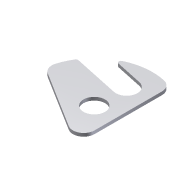
# Autodesk Inventor part: OpenROV 2_3 Dev EndCap Wire Guide
Saved by Autodesk Inventor 2012 (Build 160160000, 160)
## iProperties
Created: 2011-09-29
Part Number: OpenROV 2_3 Dev EndCap Wire Guide
Document SubType Name: Modeling
Designer: user
Density: 1 g/cm^3
Material: Default
Author: user
Autodesk Inventor part; units mm, degrees
ref_plane "YZ Plane" through (0, 0, 0) normal (1, 0, 0) x (0, 1, 0)
ref_plane "XZ Plane" through (0, 0, 0) normal (0, 1, 0) x (-1, 0, 0)
ref_plane "XY Plane" through (0, 0, 0) normal (0, 0, 1) x (1, 0, 0)
sketch "Sketch1" plane through (0, 0, 0) normal (0, 0, 1) x (1, 0, 0)
  arc A0 (-2.0957, 20.2221) -> (2.0957, 39.7779) centre (0, 30) ccw
  line L0 (2.0957, 39.7779) -> (-22.6081, 45.0726)
  line L1 (-2.0957, 20.2221) -> (-43.8855, 29.1787)
  arc A1 (12.2727, 52.5869) -> (-23.0424, 48.837) centre (0, 0) ccw
  line L2 (-47.415, 4.2576) -> (4.7008, -28.308)
  arc A2 (-46.0087, 28.2702) -> (-51.6876, 15.6331) centre (0, 0) ccw
  line L3 (20, -19.8275) -> (20, 42.8486)
  arc A3 (-23.0424, 48.837) -> (-22.6081, 45.0726) centre (-22.189, 47.0282) ccw
  arc A4 (-43.8855, 29.1787) -> (-46.0087, 28.2702) centre (-44.3047, 27.2231) ccw
  arc A5 (20, 42.8486) -> (12.2727, 52.5869) centre (10, 42.8486) ccw
  arc A6 (4.7008, -28.308) -> (20, -19.8275) centre (10, -19.8275) ccw
  arc A7 (-51.6876, 15.6331) -> (-47.415, 4.2576) centre (-42.1158, 12.7381) ccw
  circle A8 centre (0, 0) radius 10
  point P0 (-27.9334, 46.2139)
  point P1 (-45.1248, 29.4443)
  point P2 (-45.2489, 29.4709)
  point P3 (-27.9334, 46.2139)
  point P4 (20, 50.1597)
  point P5 (-53.4041, 8)
  dimension "d4" = 20
  dimension "d15" = 54
  dimension "d16" = 20
  dimension "d21" = 8
  dimension "d25" = 54
  dimension "d28" = 58
  dimension "d30" = 20
  dimension "d31" = 20
  dimension "d33" = 21.5155
  dimension "d35" = 77.903
  dimension "d36" = 2
  dimension "d37" = 10
  dimension "d38" = 30
  dimension "d41" = 20
  constraints: 22 point on circle, 11 tangent, 9 centre point, 8 end point, 7 point on line, 3 coincident, 3 equal radius, 1 parallel
  measures "d4" diameter of A0
  measures "d15" radius of A1
  measures "d16" distance between parallel lines of L0 L1
  measures "d21" vertical distance of point (0, 0) point (-53.404, 8)
  measures "d25" radius of A2
  measures "d28" angle of L3 L2
  measures "d30" distance from line of point (0, 0) L3
  measures "d31" distance from line of A0.centre L3
  measures "d33" distance from line of point (0, 0) L2
  measures "d35" angle of L3 L0
  measures "d36" radius of A3
  measures "d37" radius of A5
  measures "d38" distance of A0.centre point (0, 0)
  measures "d41" diameter of A8
extrude "Extrusion5" add sketch "Sketch1" along normal blind 3
body "Solid5"
